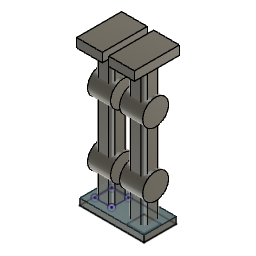
first task v2 (Autodesk Fusion 360 design; units mm, degrees)
Autodesk Fusion 360 part; units mm, degrees
sketch "Sketch1" plane through (0, 0, 0) normal (0, 0, 1) x (1, 0, 0)
  line L0 (-250, -125) -> (250, -125)
  line L1 (250, -125) -> (250, 125)
  line L2 (250, 125) -> (-250, 125)
  line L3 (-250, 125) -> (-250, -125)
  line L4 (60, 65) -> (190, 65)
  line L5 (190, 65) -> (190, -65)
  line L6 (190, -65) -> (60, -65)
  line L7 (60, -65) -> (60, 65)
  dimension "d38" = 250
  dimension "d39" = 125
  dimension "d40" = 500
  dimension "d41" = 250
  dimension "d47" = 130
  dimension "d48" = 130
  dimension "d49" = 60
  dimension "d50" = 60
  constraint horizontal L0
  constraint vertical L1
  constraint horizontal L2
  constraint vertical L3
  constraint horizontal L4
  constraint vertical L5
  constraint horizontal L6
  constraint vertical L7
  measures "d38" distance of L0 L2
  measures "d39" distance of origin L2
  measures "d40" distance of L1 L3
  measures "d41" distance of origin L1
  measures "d47" distance of L4 L6
  measures "d48" distance of L4.start L5
  measures "d49" distance of L2 L4
  measures "d50" distance of L1 L5
extrude "Extrude13" add sketch "Sketch1" along normal blind 1100 contours L4 L5 L6 L7 makes body 1
extrude "Extrude1" add sketch "Sketch1" along normal blind 50 separate body contours L0 L1 L2 L3 | L4 L5 L6 L7 makes body 2
sketch "Sketch2" plane through (0, 0, 0) normal (1, 0, 0) x (0, 1, 0)
  point P0 (250, -125)
  point P1 (250, 125)
  point P2 (-250, 125)
  point P3 (-250, -125)
  point P4 (250, -125)
  point P5 (250, 125)
  point P6 (-250, 125)
  point P7 (-250, -125)
  point P8 (-85, -65)
  point P9 (-60, -40)
  point P10 (-85, -40)
  point P11 (-60, 40)
  point P12 (-85, 65)
  point P13 (-85, 40)
  point P14 (-165, 65)
  point P15 (-190, 40)
  point P16 (-165, 40)
  point P17 (-190, -40)
  point P18 (-165, -65)
  point P19 (-165, -40)
  point P20 (250, 125)
  point P21 (-250, 125)
  point P22 (-250, -125)
  point P23 (250, -125)
  point P24 (250, -125)
  point P25 (250, 125)
sketch "Sketch3" plane through (0, 0, 50) normal (0, 0, 1) x (-1, 0, 0)
  line L0 (250, -125) -> (250, 125)
  line L1 (250, 125) -> (-250, 125)
  line L2 (-250, 125) -> (-250, -125)
  line L3 (-250, -125) -> (250, -125)
  line L4 (192.033, -65) -> (62.033, -65)
  line L5 (62.033, -65) -> (62.033, 65)
  line L6 (62.033, 65) -> (192.033, 65)
  line L7 (192.033, 65) -> (192.033, -65)
  dimension "d35" = 130
  dimension "d36" = 130
  dimension "d37" = 57.967
  dimension "d42" = 60
  constraint horizontal L4
  constraint vertical L5
  constraint horizontal L6
  constraint vertical L7
  measures "d35" distance of L5 L7
  measures "d36" distance of L4 L6
  measures "d37" distance of L0 L7
  measures "d42" distance of L3 L4
extrude "Extrude12" add sketch "Sketch3" along normal blind 1050 contours L4 L5 L6 L7 bodies 2
ref_plane "WorkPlane1" through (125, 0, 0) normal (1, 0, 0) x (0, 1, 0)
ref_plane "WorkPlane2" through (125, 0, 0) normal (1, 0, 0) x (0, 1, 0)
sketch "Sketch7" plane through (125, 0, 0) normal (1, 0, 0) x (0, 1, 0)
  circle A0 centre (0, 800) radius 100
  dimension "d14" = 200
  measures "d14" diameter of A0
extrude "Extrude4" add sketch "Sketch7" along normal blind 90 separate body makes body 3
extrude "Extrude5" add 1 faces at (125, -7.4174, 787.1527) along direction (-1, 0, 0) blind 90 on bodies 3 bodies 3
ref_plane "WorkPlane3" through (-125, 0, 0) normal (1, 0, 0) x (0, 1, 0)
sketch "Sketch9" plane through (-125, 0, 0) normal (1, 0, 0) x (0, 1, 0)
  circle A0 centre (0, 800) radius 100
  dimension "d20" = 200
  measures "d20" diameter of A0
extrude "Extrude6" add sketch "Sketch9" along normal blind 90 separate body makes body 4
extrude "Extrude7" add 1 faces at (-125, -7.4174, 787.1527) along direction (-1, 0, 0) blind 90 on bodies 4 bodies 4
sketch "Sketch10" plane through (0, 0, 0) normal (1, 0, 0) x (0, 1, 0)
ref_plane "WorkPlane4" through (125, 0, 0) normal (1, 0, 0) x (0, 1, 0)
sketch "Sketch11" plane through (125, 0, 0) normal (1, 0, 0) x (0, 1, 0)
  circle A0 centre (0, 300) radius 100
extrude "Extrude8" add sketch "Sketch11" along normal blind 90 separate body makes body 5
extrude "Extrude9" add 1 faces at (125, 12.257, 311.2936) along direction (-1, 0, 0) blind 90 on bodies 5 bodies 5
sketch "Sketch12" plane through (0, 0, 0) normal (1, 0, 0) x (0, 1, 0)
ref_plane "WorkPlane5" through (-125, 0, 0) normal (1, 0, 0) x (0, 1, 0)
sketch "Sketch13" plane through (-125, 0, 0) normal (1, 0, 0) x (0, 1, 0)
  circle A0 centre (0, 300) radius 100
extrude "Extrude10" add sketch "Sketch13" along normal blind 90 separate body makes body 6
extrude "Extrude11" add 1 faces at (-125, 12.257, 311.2936) along direction (-1, 0, 0) blind 90 on bodies 6 bodies 6
sketch "Sketch14" plane through (0, 0, 50) normal (0, 0, 1) x (-1, 0, 0)
  line L0 (250, -125) -> (250, 125)
  line L1 (250, 125) -> (-250, 125)
  line L2 (-250, 125) -> (-250, -125)
  line L3 (-250, -125) -> (250, -125)
  line L4 (192.033, 65) -> (192.033, -65)
  line L5 (192.033, -65) -> (62.033, -65)
  line L6 (62.033, -65) -> (62.033, 65)
  line L7 (62.033, 65) -> (192.033, 65)
fillet "Fillet1" radius 25 4 edges at (-192.033, -65, 575) (-62.033, -65, 575) (-192.033, 65, 575) (-62.033, 65, 575) on bodies 2
sketch "Sketch15" plane through (0, 0, 50) normal (0, 0, 1) x (1, 0, 0)
fillet "Fillet2" radius 25 4 edges at (60, -65, 550) (190, -65, 550) (190, 65, 550) (60, 65, 550) on bodies 1
sketch "Sketch16" plane through (0, 0, 1100) normal (0, 0, 1) x (-1, 0, 0)
  arc A0 (-85, -65) -> (-60, -40) centre (-85, -40) ccw
  line L0 (-60, -40) -> (-60, 40)
  arc A1 (-60, 40) -> (-85, 65) centre (-85, 40) ccw
  line L1 (-85, 65) -> (-165, 65)
  arc A2 (-165, 65) -> (-190, 40) centre (-165, 40) ccw
  line L2 (-190, 40) -> (-190, -40)
  arc A3 (-190, -40) -> (-165, -65) centre (-165, -40) ccw
  line L3 (-165, -65) -> (-85, -65)
  line L4 (-25, -175) -> (-225, -175)
  line L5 (-225, -175) -> (-225, 175)
  line L6 (-225, 175) -> (-25, 175)
  line L7 (-25, 175) -> (-25, -175)
  line L8 (250, 125) -> (-250, 125)
  line L9 (25, 175) -> (225, 175)
  line L10 (225, 175) -> (225, -175)
  line L11 (225, -175) -> (25, -175)
  line L12 (25, -175) -> (25, 175)
  line L13 (-250, -125) -> (250, -125)
  line L14 (250, -125) -> (250, 125)
  dimension "d55" = 200
  dimension "d56" = 350
  dimension "d57" = 50
  dimension "d58" = 25
  dimension "d59" = 200
  dimension "d60" = 350
  dimension "d61" = 50
  dimension "d62" = 25
  constraint horizontal L4
  constraint vertical L5
  constraint horizontal L6
  constraint vertical L7
  constraint horizontal L9
  constraint vertical L10
  constraint horizontal L11
  constraint vertical L12
  measures "d55" distance of L5 L7
  measures "d56" distance of L4 L6
  measures "d57" distance of L6 L8
  measures "d58" distance of origin L7
  measures "d59" distance of L10 L12
  measures "d60" distance of L9 L11
  measures "d61" distance of L11 L13
  measures "d62" distance of L10 L14
extrude "Extrude14" add sketch "Sketch16" along normal blind 70 contours A0 L0 A1 L1 A2 L2 A3 L3 | L4 L5 L7 L13 | L5 L7 L8 L13 | L5 L6 L7 L8 | L10 L11 L12 L13 | L8 L10 L12 L13 | L8 L9 L10 L12 bodies 1 2 4 6
